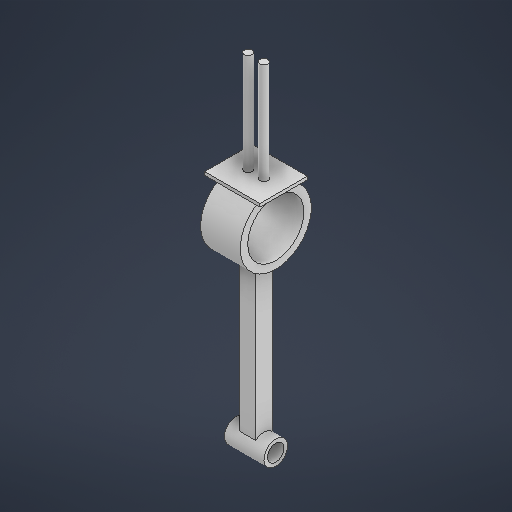
# Autodesk Inventor part: guide
Saved by Autodesk Inventor 2026.1 (Build 301233020, 233B)
## iProperties
Created: 2025-12-31
Part Number: guide
Material: Generic
Document SubType Name: Modeling
Designer: Austin Ngobeni
Density: 1 g/cm^3
Appearance: Default
Author: Austin Ngobeni
Autodesk Inventor part; units mm, degrees
ref_plane "YZ Plane" through (0, 0, 0) normal (1, 0, 0) x (0, 1, 0)
ref_plane "XZ Plane" through (0, 0, 0) normal (0, 1, 0) x (-1, 0, 0)
ref_plane "XY Plane" through (0, 0, 0) normal (0, 0, 1) x (1, 0, 0)
sketch "Sketch1" plane through (0, 0, 0) normal (1, 0, 0) x (0, 1, 0)
  circle A0 centre (0, 0) radius 5.25
  line L0 (0, 0) -> (16.2396, 0) construction
  line L1 (5.4642, 5.1373) -> (101.0943, 5.1373)
  line L2 (5.4642, -5.1373) -> (101.0943, -5.1373)
  circle A1 centre (123, 0) radius 22.5
  circle A2 centre (123, 0) radius 17.75
  circle A3 centre (0, 0) radius 7.5
  dimension "d20" = 15
  dimension "d0" = 10.5
  dimension "d14" = 45
  dimension "d16" = 35.5
  dimension "d17" = 123
  constraints: 6 end point, 4 coincident, 3 centre point, 2 horizontal, 2 point on circle, 1 horizontal alignment, 1 symmetric about line, 3 other
  measures "d0" diameter of A0
  measures "d14" diameter of A1
  measures "d16" diameter of A2
  measures "d17" distance of point (0, 0) A1.centre
extrude "Extrusion1" add sketch "Sketch1" along normal mid plane 25 contours A3 | A1
extrude "Extrusion2" add sketch "Sketch1" along normal mid plane 10 contours L1 A1 L2 A3
sketch "Sketch2" plane through (0, 0, 0) normal (0, 0, 1) x (1, 0, 0)
  line L0 (-12.5, 145.5) -> (12.5, 145.5) projected
  line L1 (0, 113.4787) -> (0, 177.5213) construction
  line L2 (-17.5, 144.5) -> (17.5, 144.5)
  line L3 (17.5, 144.5) -> (17.5, 146.5)
  line L4 (17.5, 146.5) -> (-17.5, 146.5)
  line L5 (-17.5, 146.5) -> (-17.5, 144.5)
  point P0 (0, 0)
  point P1 (0, 145.5)
  point P2 (0, 146.5)
  dimension "d21" = 1
  dimension "d22" = 2
  dimension "d23" = 35
  constraints: 10 end point, 3 midpoint, 2 parallel, 1 horizontal, 1 perpendicular, 1 vertical, 1 vertical alignment
  measures "d21" distance between parallel lines of L0 L2
  measures "d22" distance of L4.end L2.start
  measures "d23" distance of L3.end L4.end
extrude "Extrusion3" add sketch "Sketch2" along normal mid plane 30
sketch "Sketch3" plane through (-17.5, 146.5, 15) normal (0, 1, 0) x (1, 0, 0)
  circle A0 centre (22.5, 15) radius 2.5
  circle A1 centre (12.5, 15) radius 2.5
  line L0 (17.5, -7.5) -> (17.5, 37.5) construction
  line L1 (5, 37.5) -> (30, 37.5) projected
  point P0 (17.5, 15)
  dimension "d26" = 5
  dimension "d27" = 5
  dimension "d28" = 5
  dimension "d29" = 5
  constraints: 2 centre point, 2 end point, 2 midpoint
  measures "d26" diameter of A0
  measures "d27" diameter of A1
  measures "d28" distance from line of L0 A1.centre
  measures "d29" distance from line of L0 A0.centre
extrude "Extrusion4" add sketch "Sketch3" along normal blind 64
body "Solid1"
